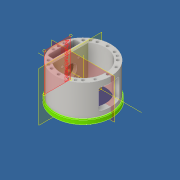
# Autodesk Inventor part: CoverBase
Saved by Autodesk Inventor 2016 (Build 200138000, 138)
## iProperties
Created: 2015-08-24
Part Number: CoverBase
Material: ABS-Kunststoff
Document SubType Name: Modeling
Designer: 4ndreas
Density: 1.06 g/cm^3
Appearance: Glatt - grün
Mass: 706.928 g
Surface Area: 1729.36 cm^2
Volume: 666.913 cm^3
Author: 4ndreas
Autodesk Inventor part; units mm, degrees
ref_plane "YZ Plane" through (0, 0, 0) normal (1, 0, 0) x (0, 1, 0)
ref_plane "XZ Plane" through (0, 0, 0) normal (0, 1, 0) x (-1, 0, 0)
ref_plane "XY Plane" through (0, 0, 0) normal (0, 0, 1) x (1, 0, 0)
sketch "Skizze1" plane through (0, 0, 0) normal (0, 0, 1) x (1, 0, 0)
  line L0 (-69.282, 40) -> (69.282, 40) projected
  arc A0 (69.282, -40) -> (80, 0) centre (0, 0) ccw projected
  arc A1 (80, 0) -> (69.282, 40) centre (0, 0) ccw projected
  circle A2 centre (-61.0246, -30) radius 2.25 projected
  circle A3 centre (-61.0246, 30) radius 2.25 projected
  circle A4 centre (68, 0) radius 2.25 projected
  circle A5 centre (61.0246, 30) radius 2.25 projected
  circle A6 centre (61.0246, -30) radius 2.25 projected
  circle A7 centre (-68, 0) radius 2.25 projected
  line L1 (59.925, 53) -> (-59.925, 53) projected
  arc A8 (59.925, 53) -> (-59.925, 53) centre (0, 0) ccw projected
  line L2 (59.925, 53) -> (-59.925, 53) projected
  arc A9 (-59.925, 53) -> (-69.282, 40) centre (0, 0) ccw projected
  line L3 (-69.282, 40) -> (69.282, 40) projected
  arc A10 (69.282, 40) -> (59.925, 53) centre (0, 0) ccw projected
  circle A11 centre (0, 0) radius 83
  line L4 (69.282, -40) -> (-69.282, -40) projected
  arc A12 (-69.282, 40) -> (-69.282, -40) centre (0, 0) ccw projected
  circle A13 centre (0, 0) radius 80
  point P0 (0, 0)
  dimension "d0" = 3
  constraints: 2 centre point, 2 coincident, 1 concentric
  measures "d0" radial gap between concentric circles of A8 A11
extrude "Extrusion1" add sketch "Skizze1" against normal blind 10 contours A11
sketch "Skizze3" plane through (0, 0, -10) normal (0, 0, -1) x (-1, 0, 0)
  circle A0 centre (0, 0) radius 83 projected
  circle A1 centre (0, 0) radius 64
  circle A2 centre (0, 0) radius 80 projected
  circle A3 centre (0, 0) radius 83 projected
  point P0 (0, 0)
  dimension "d11" = 19
  constraints: 1 centre point, 1 coincident
  measures "d11" radial gap between concentric circles of A0 A1
extrude "Extrusion2" add sketch "Skizze3" against normal blind 100 separate body contours A2
sketch "Skizze4" plane through (0, 0, -10) normal (0, 0, -1) x (-1, 0, 0)
  circle A0 centre (0, 0) radius 83 projected
  circle A1 centre (0, 0) radius 80 projected
  circle A2 centre (0, 0) radius 83 projected
  point P0 (0, 0)
extrude "Extrusion3" add sketch "Skizze4" along normal blind 5 bodies 1
fillet "Rundung1" radius 2 2 edges at (83, 0, -15) (-83, 0, 0)
sketch "Skizze6" plane through (0, 0, -10) normal (0, 0, -1) x (-1, 0, 0)
  line L0 (0, 0) -> (-67.9753, 0)
  constraints: 2 end point, 1 horizontal
ref_plane "Arbeitsebene1" through (0, 0, -10) normal (0, 1, 0) x (1, 0, 0)
sketch "Skizze8" plane through (0, 0, -10) normal (0, 0, -1) x (-1, 0, 0)
  line L0 (65, 40) -> (47, 40)
  line L1 (47, 40) -> (47, 17.5)
  line L2 (47, 17.5) -> (37, 17.5)
  line L3 (37, 17.5) -> (37, -17.5)
  line L4 (37, -17.5) -> (47, -17.5)
  line L5 (47, -17.5) -> (47, -40)
  line L6 (47, -40) -> (65, -40)
  line L7 (65, -40) -> (65, 40)
  line L8 (-3.5, -20.7707) -> (0, -22.7915)
  line L9 (0, -22.7915) -> (3.5, -20.7707)
  line L10 (3.5, -20.7707) -> (3.5, -16.7293)
  line L11 (3.5, -16.7293) -> (0, -14.7085)
  line L12 (0, -14.7085) -> (-3.5, -16.7293)
  line L13 (-3.5, -16.7293) -> (-3.5, -20.7707)
  line L14 (-3.5, 16.7293) -> (0, 14.7085)
  line L15 (0, 14.7085) -> (3.5, 16.7293)
  line L16 (3.5, 16.7293) -> (3.5, 20.7707)
  line L17 (3.5, 20.7707) -> (0, 22.7915)
  line L18 (0, 22.7915) -> (-3.5, 20.7707)
  line L19 (-3.5, 20.7707) -> (-3.5, 16.7293)
  circle A0 centre (-25, 66.453) radius 2.1
  circle A1 centre (-50, 50.4083) radius 2.1
  line L20 (10, 53.782) -> (10, 60.782)
  line L21 (10, 60.782) -> (-10, 60.782)
  line L22 (-10, 60.782) -> (-10, 53.782)
  line L23 (-10, 53.782) -> (10, 53.782)
  circle A2 centre (50, 50.4083) radius 2.1
  circle A3 centre (25, 66.453) radius 2.1
  circle A4 centre (0, 71) radius 2.1
  circle A5 centre (0, 0) radius 80
  circle A6 centre (-71, 0) radius 2.1
  circle A7 centre (-25, -66.453) radius 2.1
  circle A8 centre (-50, -50.4083) radius 2.1
  circle A9 centre (50, -50.4083) radius 2.1
  circle A10 centre (0, -71) radius 2.1
  circle A11 centre (25, -66.453) radius 2.1
  circle A12 centre (71, 0) radius 2.1
  line L24 (-10, -53.782) -> (-10, -60.782)
  line L25 (-10, -60.782) -> (10, -60.782)
  line L26 (10, -60.782) -> (10, -53.782)
  line L27 (10, -53.782) -> (-10, -53.782)
  point P0 (0, 0)
  constraints: 56 end point, 13 centre point, 12 vertical, 8 horizontal, 62 other
sketch "Skizze9" plane through (0, 0, -10) normal (0, 1, 0) x (1, 0, 0)
  arc A0 (81, -10) -> (83, -8) centre (81, -8) ccw projected
  line L0 (81, -10) -> (80, -10) projected
  line L1 (80, -10) -> (80, 5) projected
  line L2 (80, 5) -> (81, 5) projected
  arc A1 (83, 3) -> (81, 5) centre (81, 3) ccw projected
  line L3 (83, 3) -> (83, -8) projected
  arc A2 (-83, -8) -> (-81, -10) centre (-81, -8) ccw projected
  line L4 (-83, -8) -> (-83, 3) projected
  arc A3 (-81, 5) -> (-83, 3) centre (-81, 3) ccw projected
  line L5 (-81, 5) -> (-80, 5) projected
  line L6 (-80, 5) -> (-80, -10) projected
  line L7 (-80, -10) -> (-81, -10) projected
  line L8 (80, 0) -> (80, -100) projected
  line L9 (80, -100) -> (64, -100) projected
  line L10 (64, -100) -> (64, 0) projected
  line L11 (64, 0) -> (80, 0) projected
  line L12 (-80, -100) -> (-80, 0) projected
  line L13 (-80, 0) -> (-64, 0) projected
  line L14 (-64, 0) -> (-64, -100) projected
  line L15 (-64, -100) -> (-80, -100) projected
  line L16 (-104.4853, 30) -> (144.1388, 30)
  line L17 (-64, 0) -> (64, 0) projected
  line L18 (-94.4714, -53) -> (126.5007, -53)
  point P0 (0, -10)
  dimension "d13" = 30
  dimension "d14" = 83
  constraints: 4 end point, 1 horizontal, 1 parallel
  measures "d13" distance between parallel lines of L17 L16
  measures "d14" distance between parallel lines of L18 L16
ref_plane "Arbeitsebene2" through (-37, 17.5, -10) normal (1, 0, 0) x (0, -1, 0)
sketch "Skizze10" plane through (-37, 17.5, -10) normal (1, 0, 0) x (0, -1, 0)
  circle A0 centre (17.5, -53) radius 19.05
  line L0 (47.5, -83) -> (-12.5, -83)
  line L1 (-12.5, -83) -> (-12.5, -23)
  line L2 (-12.5, -23) -> (47.5, -23)
  line L3 (47.5, -23) -> (47.5, -83)
  line L4 (47.5, -83) -> (-12.5, -23) construction
  line L5 (-12.5, -83) -> (47.5, -23) construction
  line L6 (89.5555, -10) -> (88.4295, -10) projected
  line L7 (88.4295, -10) -> (88.4295, 5) projected
  line L8 (88.4295, 5) -> (89.5555, 5) projected
  line L9 (91.7967, 3) -> (91.7967, -8) projected
  line L10 (-56.7967, -8) -> (-56.7967, 3) projected
  line L11 (-54.5555, 5) -> (-53.4295, 5) projected
  line L12 (-53.4295, 5) -> (-53.4295, -10) projected
  line L13 (-53.4295, -10) -> (-54.5555, -10) projected
  line L14 (-53.4295, -100) -> (-53.4295, 0) projected
  line L15 (-53.4295, 0) -> (-34.7207, 0) projected
  line L16 (-34.7207, 0) -> (-34.7207, -100) projected
  line L17 (-34.7207, -100) -> (-53.4295, -100) projected
  line L18 (88.4295, 0) -> (88.4295, -100) projected
  line L19 (88.4295, -100) -> (69.7207, -100) projected
  line L20 (69.7207, -100) -> (69.7207, 0) projected
  line L21 (69.7207, 0) -> (88.4295, 0) projected
  line L22 (69.7207, 0) -> (-34.7207, 0)
  line L23 (69.7207, -100) -> (-34.7207, -100)
  line L24 (41.05, -76.55) -> (-6.05, -76.55) construction
  line L25 (-6.05, -76.55) -> (-6.05, -29.45) construction
  line L26 (-6.05, -29.45) -> (41.05, -29.45) construction
  line L27 (41.05, -29.45) -> (41.05, -76.55) construction
  line L28 (41.05, -76.55) -> (-6.05, -29.45) construction
  line L29 (-6.05, -76.55) -> (41.05, -29.45) construction
  circle A1 centre (41.05, -29.45) radius 2.5
  circle A2 centre (-6.05, -29.45) radius 2.5
  circle A3 centre (41.05, -76.55) radius 2.5
  circle A4 centre (-6.05, -76.55) radius 2.5
  point P0 (17.5, -10)
  dimension "d16" = 38.1
  dimension "d17" = 60
  dimension "d18" = 47.1
  dimension "d21" = 5
  constraints: 28 end point, 9 coincident, 5 centre point, 4 midpoint, 4 parallel, 3 equal radius, 3 horizontal, 3 perpendicular, 1 collinear, 1 point on line, 4 other
  measures "d16" diameter of A0
  measures "d17" distance between parallel lines of L3 L1
  measures "d18" distance between parallel lines of L27 L25
  measures "d21" diameter of A1
extrude "Extrusion4" add sketch "Skizze10" against normal blind 10 contours L0 L1 L2 L3 | L20 L23 L16 L22 bodies 2
sketch "Skizze11" plane through (-47, 17.5, -10) normal (-1, 0, 0) x (0, 0, 1)
  line L0 (10, 48.4697) -> (10, 47.2379) projected
  line L1 (10, 47.2379) -> (-5, 47.2379) projected
  line L2 (-5, 47.2379) -> (-5, 48.4697) projected
  line L3 (-3, 50.9105) -> (8, 50.9105) projected
  line L4 (8, -85.9105) -> (-3, -85.9105) projected
  line L5 (-5, -83.4697) -> (-5, -82.2379) projected
  line L6 (-5, -82.2379) -> (10, -82.2379) projected
  line L7 (10, -82.2379) -> (10, -83.4697) projected
  circle A0 centre (53, -17.5) radius 19.05 projected
  circle A1 centre (76.55, 6.05) radius 2.5 projected
  circle A2 centre (76.55, -41.05) radius 2.5 projected
  circle A3 centre (29.45, 6.05) radius 2.5 projected
  circle A4 centre (29.45, -41.05) radius 2.5 projected
  line L8 (0, -82.2379) -> (0, -60.9396) projected
  line L9 (0, -60.9396) -> (0, 25.9396) projected
  line L10 (0, 25.9396) -> (0, 47.2379) projected
  line L11 (0, 47.2379) -> (100, 47.2379) projected
  line L12 (100, 47.2379) -> (100, 25.9396) projected
  line L13 (100, 25.9396) -> (100, -60.9396) projected
  line L14 (100, -60.9396) -> (100, -82.2379) projected
  line L15 (100, -82.2379) -> (0, -82.2379) projected
  line L16 (0, -60.9396) -> (100, -60.9396) projected
  line L17 (100, 25.9396) -> (0, 25.9396) projected
  line L18 (16, -31.82) -> (16, -3.18)
  circle A5 centre (53, -17.5) radius 19.05 projected
  circle A6 centre (76.55, 6.05) radius 2.5 projected
  circle A7 centre (76.55, -41.05) radius 2.5 projected
  circle A8 centre (29.45, 6.05) radius 2.5 projected
  circle A9 centre (29.45, -41.05) radius 2.5 projected
  line L19 (-56, -17.5) -> (126, -17.5) projected
  circle A10 centre (16, -31.82) radius 2.1
  circle A11 centre (16, -3.18) radius 2.1
  line L20 (10, 48.4697) -> (10, 47.2379) projected
  line L21 (10, 47.2379) -> (-5, 47.2379) projected
  line L22 (-5, 47.2379) -> (-5, 48.4697) projected
  line L23 (-3, 50.9105) -> (8, 50.9105) projected
  line L24 (8, -85.9105) -> (-3, -85.9105) projected
  line L25 (-5, -83.4697) -> (-5, -82.2379) projected
  line L26 (-5, -82.2379) -> (10, -82.2379) projected
  line L27 (10, -82.2379) -> (10, -83.4697) projected
  line L28 (0, -82.2379) -> (0, -60.9396) projected
  line L29 (0, -60.9396) -> (0, 25.9396) projected
  line L30 (0, 25.9396) -> (0, 47.2379) projected
  line L31 (0, 47.2379) -> (100, 47.2379) projected
  line L32 (100, 47.2379) -> (100, 25.9396) projected
  line L33 (100, 25.9396) -> (100, -60.9396) projected
  line L34 (100, -60.9396) -> (100, -82.2379) projected
  line L35 (100, -82.2379) -> (0, -82.2379) projected
  line L36 (0, -60.9396) -> (100, -60.9396) projected
  line L37 (100, 25.9396) -> (0, 25.9396) projected
  point P0 (10, -17.5)
  point P1 (16, -17.5)
  dimension "d22" = 37
  dimension "d23" = 28.64
  dimension "d24" = 4.2
  constraints: 2 centre point, 2 coincident, 2 end point, 1 equal radius, 1 midpoint, 1 point on line, 1 vertical, 8 other
  measures "d22" distance from line of L18 A0.centre
  measures "d23" distance of L18.start L18.end
  measures "d24" diameter of A10
extrude "Extrusion5" cut sketch "Skizze11" along normal mid plane 100 contours A10 bodies 2
sketch "Skizze12" plane through (0, 0, -10) normal (0, 0, -1) x (-1, 0, 0)
  line L0 (65, 40) -> (47, 40) projected
  line L1 (47, -40) -> (65, -40) projected
  line L2 (47, 40) -> (65, 40)
  line L3 (65, 40) -> (65, -40)
  line L4 (65, -40) -> (47, -40)
  line L5 (47, -40) -> (47, 40)
  point P0 (0, 0)
  constraints: 8 end point, 2 parallel, 1 horizontal, 1 perpendicular
extrude "Extrusion6" cut sketch "Skizze12" against normal through all bodies 2
sketch "Skizze13" plane through (0, 0, -10) normal (0, 0, -1) x (-1, 0, 0)
  circle A0 centre (0, 0) radius 83 construction
  circle A1 centre (0, 0) radius 80 construction
  line L0 (47, 43.4396) -> (47, -43.4396) projected
  arc A2 (47, -43.4396) -> (49.96, -40) centre (0, 0) ccw projected
  line L1 (49.96, -40) -> (65, -40) projected
  line L2 (65, -40) -> (65, 40) construction
  line L3 (65, 40) -> (49.96, 40) projected
  arc A3 (49.96, 40) -> (47, 43.4396) centre (0, 0) ccw projected
  line L4 (37, -52.2207) -> (37, 52.2207) projected
  arc A4 (37, 52.2207) -> (37, -52.2207) centre (0, 0) ccw construction
  circle A5 centre (0, 0) radius 80 construction
  line L5 (47, 40) -> (49.96, 40)
  line L6 (47, -40) -> (49.96, -40)
  point P0 (0, 0)
  constraints: 4 end point, 2 point on line, 1 horizontal, 1 parallel
extrude "Extrusion7" add sketch "Skizze13" against normal up to surface (100 mm away) bodies 2
hole "Bohrung1" at (0, 71, -10) at (25, 66.453, -10) at (50, 50.4083, -10) at (71, 0, -10) at (50, -50.4083, -10) at (25, -66.453, -10) at (0, -71, -10) at (-25, -66.453, -10) at (-50, -50.4083, -10) at (-71, 0, -10) at (-50, 50.4083, -10) at (-25, 66.453, -10) direction (0, 0, 1) diameter 4.2 end through all bodies 2
fillet "Rundung2" radius 5 2 edges at (-65, 40, 40) (-65, -40, 40)
sketch "Skizze14" plane through (-47, 17.5, -10) normal (-1, 0, 0) x (0, 0, 1)
  line L0 (10, 48.4697) -> (10, 47.2379) projected
  line L1 (10, 47.2379) -> (-5, 47.2379) projected
  line L2 (-5, 47.2379) -> (-5, 48.4697) projected
  line L3 (-3, 50.9105) -> (8, 50.9105) projected
  line L4 (8, -85.9105) -> (-3, -85.9105) projected
  line L5 (-5, -83.4697) -> (-5, -82.2379) projected
  line L6 (-5, -82.2379) -> (10, -82.2379) projected
  line L7 (10, -82.2379) -> (10, -83.4697) projected
  line L8 (0, -57.5) -> (100, -57.5) projected
  line L9 (100, 22.5) -> (100, -57.5) projected
  line L10 (100, 47.2379) -> (100, 22.5) projected
  line L11 (0, 47.2379) -> (100, 47.2379) projected
  line L12 (0, 22.5) -> (0, 47.2379) projected
  line L13 (100, 22.5) -> (0, 22.5) projected
  line L14 (0, -57.5) -> (0, 22.5) projected
  line L15 (0, -82.2379) -> (0, -57.5) projected
  line L16 (100, -82.2379) -> (0, -82.2379) projected
  line L17 (100, -57.5) -> (100, -82.2379) projected
  circle A0 centre (16, -31.82) radius 2.1 projected
  circle A1 centre (53, -17.5) radius 19.05 projected
  circle A2 centre (76.55, 6.05) radius 2.5 projected
  circle A3 centre (76.55, -41.05) radius 2.5 projected
  circle A4 centre (29.45, 6.05) radius 2.5 projected
  circle A5 centre (29.45, -41.05) radius 2.5 projected
  circle A6 centre (29.45, -41.05) radius 4.5
  circle A7 centre (29.45, 6.05) radius 4.5
  circle A8 centre (76.55, 6.05) radius 4.5
  circle A9 centre (76.55, -41.05) radius 4.5
  point P0 (10, -17.5)
  dimension "d39" = 9
  constraints: 4 centre point, 4 coincident, 3 equal radius, 4 other
  measures "d39" diameter of A6
extrude "Extrusion8" cut sketch "Skizze14" along normal through all contours A2 | A3 | A4 | A5 | A6 | A7 | A8 | A9 bodies 2
sketch "Skizze15" plane through (-47, 17.5, -10) normal (-1, 0, 0) x (0, 0, 1)
  line L0 (10, 48.4697) -> (10, 47.2379) projected
  line L1 (10, 47.2379) -> (-5, 47.2379) projected
  line L2 (-5, 47.2379) -> (-5, 48.4697) projected
  line L3 (-3, 50.9105) -> (8, 50.9105) projected
  line L4 (8, -85.9105) -> (-3, -85.9105) projected
  line L5 (-5, -83.4697) -> (-5, -82.2379) projected
  line L6 (-5, -82.2379) -> (10, -82.2379) projected
  line L7 (10, -82.2379) -> (10, -83.4697) projected
  line L8 (0, -57.5) -> (100, -57.5) projected
  line L9 (100, 22.5) -> (100, -57.5) projected
  line L10 (100, 47.2379) -> (100, 22.5) projected
  line L11 (0, 47.2379) -> (100, 47.2379) projected
  line L12 (0, 22.5) -> (0, 47.2379) projected
  line L13 (100, 22.5) -> (0, 22.5) projected
  line L14 (0, -57.5) -> (0, 22.5) projected
  line L15 (0, -82.2379) -> (0, -57.5) projected
  line L16 (100, -82.2379) -> (0, -82.2379) projected
  line L17 (100, -57.5) -> (100, -82.2379) projected
  circle A0 centre (16, -31.82) radius 2.1 projected
  circle A1 centre (53, -17.5) radius 19.05 projected
  circle A2 centre (76.55, 6.05) radius 2.5 projected
  circle A3 centre (76.55, -41.05) radius 2.5 projected
  circle A4 centre (29.45, 6.05) radius 2.5 projected
  circle A5 centre (29.45, -41.05) radius 2.5 projected
  circle A6 centre (29.45, -41.05) radius 5.5
  circle A7 centre (76.55, -41.05) radius 5.5
  circle A8 centre (76.55, 6.05) radius 5.5
  circle A9 centre (29.45, 6.05) radius 5.5
  point P0 (10, -17.5)
  dimension "d42" = 11
  constraints: 4 centre point, 4 coincident, 3 equal radius, 4 other
  measures "d42" diameter of A6
extrude "Extrusion9" cut sketch "Skizze15" against normal blind 3.5 contours A2 | A3 | A4 | A5 | A6 | A7 | A8 | A9 bodies 2
sketch "Skizze16" plane through (-47, 17.5, -10) normal (-1, 0, 0) x (0, 0, 1)
  line L0 (10, 48.4697) -> (10, 47.2379) projected
  line L1 (10, 47.2379) -> (-5, 47.2379) projected
  line L2 (-5, 47.2379) -> (-5, 48.4697) projected
  line L3 (-3, 50.9105) -> (8, 50.9105) projected
  line L4 (8, -85.9105) -> (-3, -85.9105) projected
  line L5 (-5, -83.4697) -> (-5, -82.2379) projected
  line L6 (-5, -82.2379) -> (10, -82.2379) projected
  line L7 (10, -82.2379) -> (10, -83.4697) projected
  circle A0 centre (76.55, 6.05) radius 5.5 projected
  circle A1 centre (29.45, -41.05) radius 5.5 projected
  circle A2 centre (76.55, -41.05) radius 5.5 projected
  circle A3 centre (29.45, 6.05) radius 5.5 projected
  line L8 (0, -57.5) -> (100, -57.5) projected
  line L9 (100, 22.5) -> (100, -57.5) projected
  line L10 (100, 47.2379) -> (100, 22.5) projected
  line L11 (0, 47.2379) -> (100, 47.2379) projected
  line L12 (0, 22.5) -> (0, 47.2379) projected
  line L13 (100, 22.5) -> (0, 22.5) projected
  line L14 (0, -57.5) -> (0, 22.5) projected
  line L15 (0, -82.2379) -> (0, -57.5) projected
  line L16 (100, -82.2379) -> (0, -82.2379) projected
  line L17 (100, -57.5) -> (100, -82.2379) projected
  circle A4 centre (16, -31.82) radius 2.1 projected
  circle A5 centre (53, -17.5) radius 19.05 projected
  circle A6 centre (16, -31.82) radius 5
  point P0 (10, -17.5)
  dimension "d45" = 10
  constraints: 1 centre point, 1 coincident, 4 other
  measures "d45" diameter of A6
extrude "Extrusion10" add sketch "Skizze16" along normal blind 3 contours A6 bodies 2
chamfer "Fase1" distance 3 angle 45 1 edges at (-47, -14.32, 1)
sketch "Skizze17" plane through (-65, -35, -10) normal (1, 0, 0) x (0, 0, -1)
  line L0 (-10, -13.3322) -> (-10, -11.6369) projected
  line L1 (-10, -11.6369) -> (5, -11.6369) projected
  line L2 (5, -11.6369) -> (5, -13.3322) projected
  line L3 (3, -16.614) -> (-8, -16.614) projected
  line L4 (-8, 86.614) -> (3, 86.614) projected
  line L5 (5, 83.3322) -> (5, 81.6369) projected
  line L6 (5, 81.6369) -> (-10, 81.6369) projected
  line L7 (-10, 81.6369) -> (-10, 83.3322) projected
  circle A0 centre (-76.55, 58.55) radius 4.5 projected
  circle A1 centre (-29.45, 11.45) radius 4.5 projected
  circle A2 centre (-29.45, 58.55) radius 4.5 projected
  circle A3 centre (-76.55, 11.45) radius 4.5 projected
  line L8 (-100, 70) -> (0, 70) projected
  line L9 (0, 81.6369) -> (0, 70) projected
  line L10 (-100, 81.6369) -> (0, 81.6369) projected
  line L11 (-100, 70) -> (-100, 81.6369) projected
  line L12 (-100, 0) -> (-100, 70) projected
  line L13 (-100, 0) -> (0, 0) projected
  line L14 (0, 0) -> (0, -11.6369) projected
  line L15 (0, -11.6369) -> (-100, -11.6369) projected
  line L16 (-100, -11.6369) -> (-100, 0) projected
  line L17 (0, 70) -> (0, 0) projected
  circle A4 centre (-16, 20.68) radius 2.1 projected
  circle A5 centre (-16, 20.68) radius 2.1 projected
  circle A6 centre (-16, 20.68) radius 5 projected
  point P0 (-10, 35)
  constraints: 4 other
extrude "Extrusion11" add sketch "Skizze17" along normal blind 3 contours A6 bodies 2
chamfer "Fase2" distance 3 angle 45 1 edges at (-65, -14.32, 11)
ref_plane "Arbeitsebene3" through (-75, -35, -10) normal (1, 0, 0) x (0, 0, -1)
sketch "Skizze18" plane through (-75, -35, -10) normal (1, 0, 0) x (0, 0, -1)
  line L0 (-10, 4.4059) -> (-10, 7.1612) projected
  line L1 (-10, 7.1612) -> (5, 7.1612) projected
  line L2 (5, 7.1612) -> (5, 4.4059) projected
  line L3 (3, -0.5528) -> (-8, -0.5528) projected
  line L4 (-8, 70.5528) -> (3, 70.5528) projected
  line L5 (5, 65.5941) -> (5, 62.8388) projected
  line L6 (5, 62.8388) -> (-10, 62.8388) projected
  line L7 (-10, 62.8388) -> (-10, 65.5941) projected
  circle A0 centre (-16, 20.68) radius 2.1 projected
  line L8 (0, 62.8388) -> (0, 7.1612) projected
  line L9 (0, 7.1612) -> (-28.0876, 7.1612) projected
  arc A1 (-28.0876, 7.1612) -> (-30.8124, 7.1612) centre (-29.45, 11.45) ccw projected
  line L10 (-30.8124, 7.1612) -> (-75.1876, 7.1612) projected
  arc A2 (-75.1876, 7.1612) -> (-77.9124, 7.1612) centre (-76.55, 11.45) ccw projected
  line L11 (-77.9124, 7.1612) -> (-100, 7.1612) projected
  line L12 (-100, 7.1612) -> (-100, 62.8388) projected
  line L13 (-100, 62.8388) -> (-77.9124, 62.8388) projected
  arc A3 (-77.9124, 62.8388) -> (-75.1876, 62.8388) centre (-76.55, 58.55) ccw projected
  line L14 (-75.1876, 62.8388) -> (-30.8124, 62.8388) projected
  arc A4 (-30.8124, 62.8388) -> (-28.0876, 62.8388) centre (-29.45, 58.55) ccw projected
  line L15 (-28.0876, 62.8388) -> (0, 62.8388) projected
  circle A5 centre (-16, 20.68) radius 5
  point P0 (-10, 35)
  dimension "d57" = 10
  constraints: 1 centre point, 1 coincident, 4 other
  measures "d57" diameter of A5
extrude "Extrusion12" cut sketch "Skizze18" against normal through all contours A0 | A5 bodies 2
sketch "Skizze19" plane through (0, 0, 90) normal (0, 0, 1) x (1, 0, 0)
  circle A0 centre (0, 0) radius 80 projected
  circle A1 centre (-50, 50.4083) radius 2.1 projected
  circle A2 centre (-50, -50.4083) radius 2.1 projected
  circle A3 centre (0, -71) radius 2.1 projected
  circle A4 centre (50, -50.4083) radius 2.1 projected
  circle A5 centre (50, 50.4083) radius 2.1 projected
  circle A6 centre (0, 71) radius 2.1 projected
  circle A7 centre (25, 66.453) radius 2.1 projected
  circle A8 centre (71, 0) radius 2.1 projected
  circle A9 centre (25, -66.453) radius 2.1 projected
  circle A10 centre (-25, -66.453) radius 2.1 projected
  circle A11 centre (-71, 0) radius 2.1 projected
  circle A12 centre (-25, 66.453) radius 2.1 projected
  circle A13 centre (0, 0) radius 80 projected
  line L0 (-37, 52.2207) -> (-37, -52.2207) projected
  arc A14 (-37, -52.2207) -> (-37, 52.2207) centre (0, 0) ccw projected
  arc A15 (-65, -35) -> (-60, -40) centre (-60, -35) ccw projected
  line L1 (-65, -35) -> (-65, 35) projected
  arc A16 (-60, 40) -> (-65, 35) centre (-60, 35) ccw projected
  line L2 (-47, 40) -> (-60, 40) projected
  line L3 (-47, -40) -> (-47, 40) projected
  line L4 (-60, -40) -> (-47, -40) projected
  point P0 (0, 0)
hole "Bohrung2" at (25, -66.453, 90) at (0, -71, 90) at (-25, -66.453, 90) at (25, 66.453, 90) at (0, 71, 90) at (-25, 66.453, 90) direction (0, 0, -1) diameter 8 depth 47 bodies 2
sketch "Skizze20" plane through (0, 0, 90) normal (0, 0, 1) x (1, 0, 0)
  circle A0 centre (0, 71) radius 4 projected
  circle A1 centre (-25, -66.453) radius 4 projected
  circle A2 centre (25, -66.453) radius 4 projected
  circle A3 centre (0, -71) radius 4 projected
  circle A4 centre (25, 66.453) radius 4 projected
  circle A5 centre (-25, 66.453) radius 4 projected
  circle A6 centre (-50, 50.4083) radius 2.1 projected
  circle A7 centre (-50, -50.4083) radius 2.1 projected
  circle A8 centre (50, -50.4083) radius 2.1 projected
  circle A9 centre (50, 50.4083) radius 2.1 projected
  circle A10 centre (71, 0) radius 2.1 projected
  circle A11 centre (-71, 0) radius 2.1 projected
  circle A12 centre (0, 0) radius 80 projected
  line L0 (-37, 52.2207) -> (-37, -52.2207) projected
  arc A13 (-37, -52.2207) -> (-37, 52.2207) centre (0, 0) ccw projected
  arc A14 (-65, -35) -> (-60, -40) centre (-60, -35) ccw projected
  line L1 (-65, -35) -> (-65, 35) projected
  arc A15 (-60, 40) -> (-65, 35) centre (-60, 35) ccw projected
  line L2 (-47, 40) -> (-60, 40) projected
  line L3 (-47, -40) -> (-47, 40) projected
  line L4 (-60, -40) -> (-47, -40) projected
  point P0 (0, 0)
hole "Bohrung3" at (50, -50.4083, 90) at (71, 0, 90) at (50, 50.4083, 90) at (-50, 50.4083, 90) at (-71, 0, 90) at (-50, -50.4083, 90) direction (0, 0, -1) diameter 8 depth 52 bodies 2
sketch "Skizze21" plane through (0, 0, -10) normal (0, 0, -1) x (-1, 0, 0)
  circle A0 centre (0, 0) radius 83 projected
  circle A1 centre (0, 0) radius 80 projected
  line L0 (47, 40) -> (47, -40) projected
  line L1 (47, -40) -> (60, -40) projected
  arc A2 (60, -40) -> (65, -35) centre (60, -35) ccw projected
  line L2 (65, -35) -> (65, 35) projected
  arc A3 (65, 35) -> (60, 40) centre (60, 35) ccw projected
  line L3 (60, 40) -> (47, 40) projected
  circle A4 centre (50, 50.4083) radius 2.1 projected
  circle A5 centre (50, -50.4083) radius 2.1 projected
  circle A6 centre (0, -71) radius 2.1 projected
  circle A7 centre (-50, -50.4083) radius 2.1 projected
  circle A8 centre (-50, 50.4083) radius 2.1 projected
  circle A9 centre (0, 71) radius 2.1 projected
  circle A10 centre (-25, 66.453) radius 2.1 projected
  circle A11 centre (-71, 0) radius 2.1 projected
  circle A12 centre (-25, -66.453) radius 2.1 projected
  circle A13 centre (25, -66.453) radius 2.1 projected
  circle A14 centre (71, 0) radius 2.1 projected
  circle A15 centre (25, 66.453) radius 2.1 projected
  line L4 (37, -52.2207) -> (37, 52.2207) projected
  arc A16 (37, 52.2207) -> (37, -52.2207) centre (0, 0) ccw projected
  circle A17 centre (0, 0) radius 80 projected
  line L5 (-62.9361, 27.118) -> (-66.9622, 26.7657)
  line L6 (-66.9622, 26.7657) -> (-69.2802, 30.0763)
  line L7 (-69.2802, 30.0763) -> (-67.5722, 33.7391)
  line L8 (-67.5722, 33.7391) -> (-63.5462, 34.0913)
  line L9 (-63.5462, 34.0913) -> (-61.2281, 30.7808)
  line L10 (-61.2281, 30.7808) -> (-62.9361, 27.118)
  line L11 (0, 0) -> (-65.2542, 30.4285) construction
  line L12 (0, 0) -> (-71, 0) construction
  line L13 (-58.0037, 27.0476) -> (-72.5046, 33.8095) construction
  circle A18 centre (-65.2542, 30.4285) radius 2.1
  line L14 (0, 0) -> (38.8886, 60.5943) construction
  line L15 (0, 0) -> (70.2933, 15.5837) construction
  line L16 (0, 0) -> (-38.8886, 60.5943) construction
  line L17 (-25, 66.453) -> (-50, 50.4083) construction
  line L18 (25, 66.453) -> (50, 50.4083) construction
  line L19 (71, 0) -> (0, 0) construction
  line L20 (-35.2976, 58.7402) -> (-38.6988, 56.5574)
  line L21 (-38.6988, 56.5574) -> (-42.2899, 58.4115)
  line L22 (-42.2899, 58.4115) -> (-42.4797, 62.4485)
  line L23 (-42.4797, 62.4485) -> (-39.0784, 64.6313)
  line L24 (-39.0784, 64.6313) -> (-35.4874, 62.7772)
  line L25 (-35.4874, 62.7772) -> (-35.2976, 58.7402)
  line L26 (39.0784, 64.6313) -> (42.4797, 62.4485)
  line L27 (42.4797, 62.4485) -> (42.2899, 58.4115)
  line L28 (42.2899, 58.4115) -> (38.6988, 56.5574)
  line L29 (38.6988, 56.5574) -> (35.2976, 58.7402)
  line L30 (35.2976, 58.7402) -> (35.4874, 62.7772)
  line L31 (35.4874, 62.7772) -> (39.0784, 64.6313)
  line L32 (66.4389, 16.7989) -> (69.4186, 19.5293)
  line L33 (69.4186, 19.5293) -> (73.273, 18.314)
  line L34 (73.273, 18.314) -> (74.1477, 14.3684)
  line L35 (74.1477, 14.3684) -> (71.168, 11.638)
  line L36 (71.168, 11.638) -> (67.3136, 12.8533)
  line L37 (67.3136, 12.8533) -> (66.4389, 16.7989)
  circle A19 centre (-38.8886, 60.5943) radius 2.1
  circle A20 centre (38.8886, 60.5943) radius 2.1
  circle A21 centre (70.2933, 15.5837) radius 2.1
  circle A22 centre (-65.2542, 30.4285) radius 5
  circle A23 centre (-38.8886, 60.5943) radius 5
  circle A24 centre (38.8886, 60.5943) radius 5
  circle A25 centre (70.2933, 15.5837) radius 5
  point P0 (0, 0)
  point P1 (-37.5, 58.4307)
  point P2 (37.5, 58.4307)
  dimension "d74" = 25
  dimension "d75" = 7
  dimension "d78" = 4.2
  dimension "d82" = 12.5
  dimension "d83" = 10
  constraints: 66 end point, 11 coincident, 8 centre point, 6 equal length, 6 equal radius, 4 perpendicular, 3 midpoint, 3 point on line, 2 horizontal, 1 point on circle, 54 other
  measures "d74" angle of L12 L11
  measures "d75" distance between parallel lines of L10 L7
  measures "d78" diameter of A18
  measures "d82" angle of L15 L19
  measures "d83" diameter of A22
extrude "Extrusion13" cut sketch "Skizze21" against normal blind 16 contours L5 L6 L7 L8 L9 L10 | A18 | L20 L21 L22 L23 L24 L25 | L26 L27 L28 L29 L30 L31 | L32 L33 L34 L35 L36 L37 | A19 | A20 | A21 | A22 | A23 | A24 | A25 bodies 2
extrude "Extrusion14" cut sketch "Skizze21" against normal through all contours A18 | A19 | A20 | A21 bodies 2
mirror "Spiegeln1" about plane through (0, 0, -10) normal (0, 1, 0) of "Extrusion14", "Extrusion13" bodies 2
sketch "Skizze23" plane through (0, 0, 90) normal (0, 0, 1) x (1, 0, 0)
  circle A0 centre (-70.2933, -15.5837) radius 2.1 projected
  circle A1 centre (38.8886, -60.5943) radius 2.1 projected
  circle A2 centre (65.2542, -30.4285) radius 2.1 projected
  circle A3 centre (-38.8886, -60.5943) radius 2.1 projected
  circle A4 centre (-38.8886, 60.5943) radius 2.1 projected
  circle A5 centre (65.2542, 30.4285) radius 2.1 projected
  circle A6 centre (38.8886, 60.5943) radius 2.1 projected
  circle A7 centre (-70.2933, 15.5837) radius 2.1 projected
  circle A8 centre (-71, 0) radius 4 projected
  circle A9 centre (50, 50.4083) radius 4 projected
  circle A10 centre (50, -50.4083) radius 4 projected
  circle A11 centre (71, 0) radius 4 projected
  circle A12 centre (-50, 50.4083) radius 4 projected
  circle A13 centre (-50, -50.4083) radius 4 projected
  circle A14 centre (0, 71) radius 4 projected
  circle A15 centre (-25, -66.453) radius 4 projected
  circle A16 centre (25, -66.453) radius 4 projected
  circle A17 centre (0, -71) radius 4 projected
  circle A18 centre (25, 66.453) radius 4 projected
  circle A19 centre (-25, 66.453) radius 4 projected
  line L0 (-47, -40) -> (-47, 40) projected
  line L1 (-47, 40) -> (-60, 40) projected
  arc A20 (-60, 40) -> (-65, 35) centre (-60, 35) ccw projected
  line L2 (-65, 35) -> (-65, -35) projected
  arc A21 (-65, -35) -> (-60, -40) centre (-60, -35) ccw projected
  line L3 (-60, -40) -> (-47, -40) projected
  line L4 (-37, 52.2207) -> (-37, -52.2207) projected
  arc A22 (-37, -52.2207) -> (-37, 52.2207) centre (0, 0) ccw projected
  circle A23 centre (0, 0) radius 80 projected
  line L5 (63.5462, -34.0913) -> (61.2281, -30.7808)
  line L6 (61.2281, -30.7808) -> (62.9361, -27.118)
  line L7 (62.9361, -27.118) -> (66.9622, -26.7657)
  line L8 (66.9622, -26.7657) -> (69.2802, -30.0763)
  line L9 (69.2802, -30.0763) -> (67.5722, -33.7391)
  line L10 (67.5722, -33.7391) -> (63.5462, -34.0913)
  line L11 (35.4874, -62.7772) -> (35.2976, -58.7402)
  line L12 (35.2976, -58.7402) -> (38.6988, -56.5574)
  line L13 (38.6988, -56.5574) -> (42.2899, -58.4115)
  line L14 (42.2899, -58.4115) -> (42.4797, -62.4485)
  line L15 (42.4797, -62.4485) -> (39.0784, -64.6313)
  line L16 (39.0784, -64.6313) -> (35.4874, -62.7772)
  line L17 (-42.2899, -58.4115) -> (-38.6988, -56.5574)
  line L18 (-38.6988, -56.5574) -> (-35.2976, -58.7402)
  line L19 (-35.2976, -58.7402) -> (-35.4874, -62.7772)
  line L20 (-35.4874, -62.7772) -> (-39.0784, -64.6313)
  line L21 (-39.0784, -64.6313) -> (-42.4797, -62.4485)
  line L22 (-42.4797, -62.4485) -> (-42.2899, -58.4115)
  line L23 (-71.168, -11.638) -> (-67.3136, -12.8533)
  line L24 (-67.3136, -12.8533) -> (-66.4389, -16.7989)
  line L25 (-66.4389, -16.7989) -> (-69.4186, -19.5293)
  line L26 (-69.4186, -19.5293) -> (-73.273, -18.314)
  line L27 (-73.273, -18.314) -> (-74.1477, -14.3684)
  line L28 (-74.1477, -14.3684) -> (-71.168, -11.638)
  line L29 (65.2542, -30.4285) -> (0, 0) construction
  line L30 (0, 0) -> (-70.2933, -15.5837) construction
  line L31 (38.8886, -60.5943) -> (0, 0) construction
  line L32 (-38.8886, -60.5943) -> (0, 0) construction
  point P0 (0, 0)
  dimension "d84" = 7
  constraints: 56 end point, 4 coincident, 4 perpendicular, 3 equal length, 52 other
  measures "d84" distance between parallel lines of L7 L10
extrude "Extrusion15" cut sketch "Skizze23" against normal blind 20 contours A0 | A1 | A2 | A3 | L5 L6 L7 L8 L9 L10 | L11 L12 L13 L14 L15 L16 | L17 L18 L19 L20 L21 L22 | L23 L24 L25 L26 L27 L28 bodies 2
mirror "Spiegeln2" about plane through (0, 0, -10) normal (0, 1, 0) of "Extrusion15" bodies 2
sketch "Skizze24" plane through (-75, -35, -10) normal (-1, 0, 0) x (0, 0, 1)
  arc A0 (11.9637, 17.729) -> (11.018, 21.1037) centre (16, 20.68) ccw projected
  line L0 (16, 14.4163) -> (0, 14.4163) projected
  spline S0 degree 2 poles (11, 20.68) (11, 29.3403) (18.5, 25.0101) (26, 20.68) (18.5, 16.3499) (11, 12.0197) (11, 20.68) knots 0 0 0 0.333333 0.333333 0.666667 0.666667 1 1 1 weights 1 0.5 1 0.5 1 0.5 1 projected
  point P0 (10, 35)
  constraints: 1 other
extrude "Extrusion16" add sketch "Skizze24" against normal up to surface (13 mm away) bodies 2
sketch "Skizze26" plane through (-75, -35, -10) normal (-1, 0, 0) x (0, 0, 1)
  arc A0 (11.9637, 17.729) -> (11.018, 21.1037) centre (16, 20.68) ccw projected
  spline S0 degree 2 poles (11.018, 21.1037) (11, 20.8922) (11, 20.68) (11, 19.0471) (11.9637, 17.729) knots 0 0 0 0.131025 0.131025 1 1 1 weights 0.95445 0.976081 1 0.841365 0.78339 projected
  point P0 (10, 35)
  constraints: 1 other
extrude "Extrusion18" add sketch "Skizze26" along normal blind 2 bodies 2
sketch "Skizze25" plane through (0, 0, -10) normal (0, 0, -1) x (-1, 0, 0)
  circle A0 centre (70.2933, -15.5837) radius 5 projected
  point P0 (0, 0)
extrude "Extrusion17" add sketch "Skizze25" against normal blind 25 bodies 2
sketch "Skizze27" plane through (0, 0, -10) normal (0, 0, -1) x (-1, 0, 0)
  circle A0 centre (70.2933, -15.5837) radius 2.1 projected
  circle A1 centre (70.2933, -15.5837) radius 2.1 projected
  circle A2 centre (70.2933, -15.5837) radius 3.5
  point P0 (0, 0)
  dimension "d93" = 7
  constraints: 1 centre point, 1 coincident
  measures "d93" diameter of A2
extrude "Extrusion19" cut sketch "Skizze27" against normal blind 25 contours A0 | A2 bodies 2
sketch "Skizze28" plane through (-37, 17.5, -10) normal (1, 0, 0) x (0, 0, -1)
  circle A0 centre (-16, -31.82) radius 2.1 projected
  circle A1 centre (-16, -31.82) radius 2.1 projected
  point P0 (-10, -17.5)
extrude "Extrusion20" cut sketch "Skizze28" against normal through all bodies 2
sketch "Skizze29" plane through (0, 0, 90) normal (0, 0, 1) x (1, 0, 0)
  line L0 (-42.2899, 58.4115) -> (-42.4797, 62.4485) projected
  line L1 (-42.4797, 62.4485) -> (-39.0784, 64.6313) projected
  line L2 (-39.0784, 64.6313) -> (-35.4874, 62.7772) projected
  line L3 (-35.4874, 62.7772) -> (-35.2976, 58.7402) projected
  line L4 (-35.2976, 58.7402) -> (-38.6988, 56.5574) projected
  line L5 (-38.6988, 56.5574) -> (-42.2899, 58.4115) projected
  line L6 (63.5462, 34.0913) -> (67.5722, 33.7391) projected
  line L7 (67.5722, 33.7391) -> (69.2802, 30.0763) projected
  line L8 (69.2802, 30.0763) -> (66.9622, 26.7657) projected
  line L9 (66.9622, 26.7657) -> (62.9361, 27.118) projected
  line L10 (62.9361, 27.118) -> (61.2281, 30.7808) projected
  line L11 (61.2281, 30.7808) -> (63.5462, 34.0913) projected
  line L12 (35.4874, 62.7772) -> (39.0784, 64.6313) projected
  line L13 (39.0784, 64.6313) -> (42.4797, 62.4485) projected
  line L14 (42.4797, 62.4485) -> (42.2899, 58.4115) projected
  line L15 (42.2899, 58.4115) -> (38.6988, 56.5574) projected
  line L16 (38.6988, 56.5574) -> (35.2976, 58.7402) projected
  line L17 (35.2976, 58.7402) -> (35.4874, 62.7772) projected
  line L18 (-71.168, 11.638) -> (-74.1477, 14.3684) projected
  line L19 (-74.1477, 14.3684) -> (-73.273, 18.314) projected
  line L20 (-73.273, 18.314) -> (-69.4186, 19.5293) projected
  line L21 (-69.4186, 19.5293) -> (-66.4389, 16.7989) projected
  line L22 (-66.4389, 16.7989) -> (-67.3136, 12.8533) projected
  line L23 (-67.3136, 12.8533) -> (-71.168, 11.638) projected
  line L24 (-42.4797, -62.4485) -> (-42.2899, -58.4115) projected
  line L25 (-42.2899, -58.4115) -> (-38.6988, -56.5574) projected
  line L26 (-38.6988, -56.5574) -> (-35.2976, -58.7402) projected
  line L27 (-35.2976, -58.7402) -> (-35.4874, -62.7772) projected
  line L28 (-35.4874, -62.7772) -> (-39.0784, -64.6313) projected
  line L29 (-39.0784, -64.6313) -> (-42.4797, -62.4485) projected
  line L30 (67.5722, -33.7391) -> (63.5462, -34.0913) projected
  line L31 (63.5462, -34.0913) -> (61.2281, -30.7808) projected
  line L32 (61.2281, -30.7808) -> (62.9361, -27.118) projected
  line L33 (62.9361, -27.118) -> (66.9622, -26.7657) projected
  line L34 (66.9622, -26.7657) -> (69.2802, -30.0763) projected
  line L35 (69.2802, -30.0763) -> (67.5722, -33.7391) projected
  line L36 (39.0784, -64.6313) -> (35.4874, -62.7772) projected
  line L37 (35.4874, -62.7772) -> (35.2976, -58.7402) projected
  line L38 (35.2976, -58.7402) -> (38.6988, -56.5574) projected
  line L39 (38.6988, -56.5574) -> (42.2899, -58.4115) projected
  line L40 (42.2899, -58.4115) -> (42.4797, -62.4485) projected
  line L41 (42.4797, -62.4485) -> (39.0784, -64.6313) projected
  line L42 (-74.1477, -14.3684) -> (-71.168, -11.638) projected
  line L43 (-71.168, -11.638) -> (-67.3136, -12.8533) projected
  line L44 (-67.3136, -12.8533) -> (-66.4389, -16.7989) projected
  line L45 (-66.4389, -16.7989) -> (-69.4186, -19.5293) projected
  line L46 (-69.4186, -19.5293) -> (-73.273, -18.314) projected
  line L47 (-73.273, -18.314) -> (-74.1477, -14.3684) projected
  circle A0 centre (-71, 0) radius 4 projected
  circle A1 centre (50, 50.4083) radius 4 projected
  circle A2 centre (50, -50.4083) radius 4 projected
  circle A3 centre (71, 0) radius 4 projected
  circle A4 centre (-50, 50.4083) radius 4 projected
  circle A5 centre (-50, -50.4083) radius 4 projected
  circle A6 centre (0, 71) radius 4 projected
  circle A7 centre (-25, -66.453) radius 4 projected
  circle A8 centre (25, -66.453) radius 4 projected
  circle A9 centre (0, -71) radius 4 projected
  circle A10 centre (25, 66.453) radius 4 projected
  circle A11 centre (-25, 66.453) radius 4 projected
  line L48 (-47, 40) -> (-60, 40) projected
  line L49 (-47, -40) -> (-47, 40) projected
  line L50 (-60, -40) -> (-47, -40) projected
  arc A12 (-65, -35) -> (-60, -40) centre (-60, -35) ccw projected
  line L51 (-65, -35) -> (-65, 35) projected
  arc A13 (-60, 40) -> (-65, 35) centre (-60, 35) ccw projected
  line L52 (-37, 52.2207) -> (-37, -52.2207) projected
  arc A14 (-37, -52.2207) -> (-37, 52.2207) centre (0, 0) ccw projected
  circle A15 centre (0, 0) radius 80 projected
  line L53 (-37, 31) -> (63, 31)
  line L54 (63, 31) -> (63, -31)
  line L55 (63, -31) -> (-37, -31)
  line L56 (-37, -31) -> (-37, 31)
  line L57 (-71, 0) -> (71, 0) construction
  point P0 (0, 0)
  dimension "d98" = 100
  dimension "d99" = 62
  constraints: 10 end point, 2 horizontal, 2 parallel, 1 perpendicular, 1 point on line, 1 other
  measures "d98" distance between parallel lines of L52 L54
  measures "d99" distance between parallel lines of L55 L53
sketch "Skizze30" plane through (-37, 17.5, -10) normal (1, 0, 0) x (0, 0, -1)
  line L0 (-10, -89.5555) -> (-10, -88.4295) projected
  line L1 (-10, -88.4295) -> (5, -88.4295) projected
  line L2 (5, -88.4295) -> (5, -89.5555) projected
  line L3 (3, -91.7967) -> (-8, -91.7967) projected
  line L4 (-8, 56.7967) -> (3, 56.7967) projected
  line L5 (5, 54.5555) -> (5, 53.4295) projected
  line L6 (5, 53.4295) -> (-10, 53.4295) projected
  line L7 (-10, 53.4295) -> (-10, 54.5555) projected
  line L8 (-16, -82.7239) -> (0, -82.7239) projected
  line L9 (0, -82.7239) -> (0, -88.4295) projected
  line L10 (0, -88.4295) -> (-100, -88.4295) projected
  line L11 (-100, -88.4295) -> (-100, -81.0582) projected
  line L12 (-100, -81.0582) -> (-80, -81.0582) projected
  line L13 (-80, -81.0582) -> (-80, -79.0126) projected
  line L14 (-80, -79.0126) -> (-16, -79.0126) projected
  line L15 (-16, -79.0126) -> (-16, -82.7239) projected
  line L16 (0, 47.7239) -> (-16, 47.7239) projected
  line L17 (-16, 47.7239) -> (-16, 44.0126) projected
  line L18 (-16, 44.0126) -> (-80, 44.0126) projected
  line L19 (-80, 44.0126) -> (-80, 46.0582) projected
  line L20 (-80, 46.0582) -> (-100, 46.0582) projected
  line L21 (-100, 46.0582) -> (-100, 53.4295) projected
  line L22 (-100, 53.4295) -> (0, 53.4295) projected
  line L23 (0, 53.4295) -> (0, 47.7239) projected
  line L24 (-16, 38.4648) -> (0, 38.4648) projected
  line L25 (0, 38.4648) -> (0, 34.7207) projected
  line L26 (0, 34.7207) -> (0, -69.7207) projected
  line L27 (0, -69.7207) -> (0, -73.4648) projected
  line L28 (0, -73.4648) -> (-16, -73.4648) projected
  line L29 (-16, -73.4648) -> (-16, -77.1761) projected
  line L30 (-16, -77.1761) -> (-80, -77.1761) projected
  line L31 (-80, -77.1761) -> (-80, -75.1476) projected
  line L32 (-80, -75.1476) -> (-100, -75.1476) projected
  line L33 (-100, -75.1476) -> (-100, -69.7207) projected
  line L34 (-100, -69.7207) -> (-100, 34.7207) projected
  line L35 (-100, 34.7207) -> (-100, 40.1476) projected
  line L36 (-100, 40.1476) -> (-80, 40.1476) projected
  line L37 (-80, 40.1476) -> (-80, 42.1761) projected
  line L38 (-80, 42.1761) -> (-16, 42.1761) projected
  line L39 (-16, 42.1761) -> (-16, 38.4648) projected
  line L40 (0, 34.7207) -> (-100, 34.7207) projected
  line L41 (-100, -69.7207) -> (0, -69.7207) projected
  circle A0 centre (-16, -31.82) radius 2.1 projected
  circle A1 centre (-53, -17.5) radius 19.05 projected
  circle A2 centre (-76.55, 6.05) radius 2.5 projected
  circle A3 centre (-76.55, -41.05) radius 2.5 projected
  circle A4 centre (-29.45, 6.05) radius 2.5 projected
  circle A5 centre (-29.45, -41.05) radius 2.5 projected
  line L42 (-77, 12.5) -> (-29, 12.5)
  line L43 (-23, 6.5) -> (-23, -41.5)
  line L44 (-29, -47.5) -> (-77, -47.5)
  line L45 (-83, -41.5) -> (-83, 6.5)
  line L46 (-83, 12.5) -> (-23, -47.5) construction
  line L47 (-23, 12.5) -> (-83, -47.5) construction
  arc A6 (-23, 6.5) -> (-29, 12.5) centre (-29, 6.5) ccw
  arc A7 (-29, -47.5) -> (-23, -41.5) centre (-29, -41.5) ccw
  arc A8 (-77, 12.5) -> (-83, 6.5) centre (-77, 6.5) ccw
  arc A9 (-83, -41.5) -> (-77, -47.5) centre (-77, -41.5) ccw
  point P0 (-10, -17.5)
  dimension "d100" = 60
  dimension "d103" = 6
  constraints: 12 end point, 9 point on line, 8 point on circle, 8 tangent, 4 centre point, 3 equal radius, 2 midpoint, 2 parallel, 1 horizontal, 1 perpendicular, 4 other
  measures "d100" distance between parallel lines of L45 L43
  measures "d103" radius of A6
extrude "Extrusion21" cut sketch "Skizze30" along normal blind 120 contours A1 | A2 | A3 | A4 | A5 | L42 A6 L43 A7 L44 A9 L45 A8 bodies 2
sketch "Skizze32" plane through (59.3296, -24, 13) normal (0, 0, 1) x (1, 0, 0)
  circle A0 centre (11.6704, 24) radius 4 projected
  point P0 (-59.3296, 24)
extrude "Extrusion23" cut sketch "Skizze32" against normal blind 6 bodies 2
sketch "Skizze33" plane through (71, 0, 7) normal (0, 0, 1) x (1, 0, 0)
  circle A0 centre (0, 0) radius 2.1 projected
  point P0 (-71, 0)
extrude "Extrusion24" add sketch "Skizze33" against normal blind 0.2 bodies 2
sketch "Skizze34" plane through (59.3296, -24, 13) normal (0, 0, 1) x (1, 0, 0)
  circle A0 centre (11.6704, 24) radius 4 projected
  point P0 (-59.3296, 24)
extrude "Extrusion25" add sketch "Skizze34" against normal blind 0.2 bodies 2
sketch "Skizze35" plane through (-71, 0, 38) normal (0, 0, 1) x (1, 0, 0)
  circle A0 centre (0, 0) radius 2.1 projected
  circle A1 centre (0, 0) radius 4 projected
  point P0 (71, 0)
  dimension "d114" = 145
  dimension "d115" = 150
extrude "Extrusion26" add sketch "Skizze35" along normal blind 4 bodies 2
sketch "Skizze31" plane through (59.3296, -24, 13) normal (0, 0, 1) x (1, 0, 0)
  circle A0 centre (5.9246, 54.4285) radius 2.1 projected
  circle A1 centre (-129.6229, 8.4163) radius 3.5 projected
  circle A2 centre (-20.441, -36.5943) radius 2.1 projected
  circle A3 centre (5.9246, -6.4285) radius 2.1 projected
  circle A4 centre (-98.2182, -36.5943) radius 2.1 projected
  circle A5 centre (-98.2182, 84.5943) radius 2.1 projected
  circle A6 centre (-20.441, 84.5943) radius 2.1 projected
  circle A7 centre (-129.6229, 39.5837) radius 2.1 projected
  line L0 (-106.3296, 13.553) -> (-106.3296, 64) projected
  line L1 (-106.3296, 64) -> (-119.3296, 64) projected
  arc A8 (-119.3296, 64) -> (-124.3296, 59) centre (-119.3296, 59) ccw projected
  line L2 (-124.3296, 59) -> (-124.3296, 13.553) projected
  line L3 (-124.3296, 5.807) -> (-124.3296, -11) projected
  arc A9 (-124.3296, -11) -> (-119.3296, -16) centre (-119.3296, -11) ccw projected
  line L4 (-119.3296, -16) -> (-106.3296, -16) projected
  line L5 (-106.3296, -16) -> (-106.3296, 5.807) projected
  circle A10 centre (-109.3296, 74.4083) radius 2.1 projected
  circle A11 centre (-109.3296, -26.4083) radius 2.1 projected
  circle A12 centre (-59.3296, -47) radius 2.1 projected
  circle A13 centre (-9.3296, -26.4083) radius 2.1 projected
  circle A14 centre (-9.3296, 74.4083) radius 2.1 projected
  circle A15 centre (-59.3296, 95) radius 2.1 projected
  circle A16 centre (-34.3296, 90.453) radius 2.1 projected
  circle A17 centre (11.6704, 24) radius 2.1 projected
  circle A18 centre (-34.3296, -42.453) radius 2.1 projected
  circle A19 centre (-84.3296, -42.453) radius 2.1 projected
  circle A20 centre (-130.3296, 24) radius 2.1 projected
  circle A21 centre (-84.3296, 90.453) radius 2.1 projected
  line L6 (-96.3296, 76.2207) -> (-96.3296, -28.2207) projected
  arc A22 (-96.3296, -28.2207) -> (0, 0) centre (-59.3296, 24) ccw projected
  line L7 (16.9855, 0) -> (0, 0) projected
  arc A23 (16.9855, 0) -> (16.9855, 48) centre (-59.3296, 24) ccw projected
  line L8 (16.9855, 48) -> (0, 48) projected
  arc A24 (0, 0) -> (0, 48) centre (-59.3296, 24) ccw projected
  arc A25 (0, 48) -> (-96.3296, 76.2207) centre (-59.3296, 24) ccw projected
  arc A26 (16.9855, 48) -> (16.9855, 0) centre (-59.3296, 24) ccw projected
  point P0 (-59.3296, 24)
  constraints: 2 vertical alignment
